vrholder (Autodesk Fusion 360 design; units mm, degrees)
Autodesk Fusion 360 part; units mm, degrees
sketch "Sketch1" plane through (0, 0, 0) normal (1, 0, 0) x (0, 1, 0)
  line L0 (0, 0) -> (0, -40)
  line L1 (0, -40) -> (18.2, -40)
  line L2 (18.2, -40) -> (18.2, 30)
  line L3 (18.2, 30) -> (27.2, 30)
  line L4 (27.2, 30) -> (27.2, 48.65)
  line L5 (33.2, 48.6647) -> (77.2, 48.6647)
  line L6 (77.2, 48.6647) -> (77.2, 68.6647)
  line L7 (27.2, 48.65) -> (7.2, 48.65)
  line L8 (0, 0) -> (-8, 0)
  line L9 (-8, 0) -> (-8, -48)
  line L10 (-8, -48) -> (24.2, -48)
  line L11 (24.2, -48) -> (24.2, 2.6994)
  line L12 (33.2, 22) -> (33.2, 40.6647)
  line L13 (33.2, 40.6647) -> (33.2, 48.6647)
  line L14 (7.2, 48.65) -> (7.2, 54.65)
  line L15 (7.2, 54.65) -> (71.2, 54.65)
  line L16 (71.2, 54.65) -> (71.2, 68.6647)
  line L17 (71.2, 68.6647) -> (77.2, 68.6647)
  line L18 (33.2, 22) -> (24.2, 2.6994)
  line L19 (77.2, 48.6647) -> (24.2, -48)
  line L20 (70.3573, 48.6647) -> (24.2, -35.5199)
  line L21 (33.2, 40.6647) -> (39.2, 48.6647)
  dimension "d1" = 40
  dimension "d2" = 18.2
  dimension "d3" = 70
  dimension "d4" = 9
  dimension "d5" = 18.65
  dimension "d6" = 50
  dimension "d7" = 20
  dimension "d8" = 20
  dimension "d9" = 8
  dimension "d10" = 8
  dimension "d11" = 6
  dimension "d13" = 6
  dimension "d14" = 25
  dimension "d15" = 8
  dimension "d16" = 6
  dimension "d17" = 6
  dimension "d18" = 44
  dimension "d21" = 6
  dimension "d22" = 6
  dimension "d23" = 8
  constraint coincident L0.start L8.start
  constraint vertical L0
  constraint perpendicular L0 L1
  constraint perpendicular L1 L2
  constraint perpendicular L2 L3
  constraint perpendicular L3 L4
  constraint perpendicular L4 L5
  constraint perpendicular L5 L6
  constraint perpendicular L4 L7
  constraint perpendicular L0 L8
  constraint perpendicular L8 L9
  constraint perpendicular L0 L10
  constraint perpendicular L10 L11
  constraint perpendicular L5 L13
  constraint perpendicular L7 L14
  constraint perpendicular L14 L15
  constraint perpendicular L15 L16
  constraint parallel L5 L17
  constraint coincident L5 L20.start
  constraint coincident L11 L20.end
  constraint parallel L19 L20
  constraint coincident L5 L21.end
  measures "d1" distance of L0.start L0.end
  measures "d2" distance of L0.end L1.end
  measures "d3" distance of L1.end L2.end
  measures "d4" distance of L2.end L3.end
  measures "d5" distance of L3.end L4.end
  measures "d6" distance of L4.end L5.end
  measures "d7" distance of L5.end L6.end
  measures "d8" distance of L4.end L7.end
  measures "d9" distance of L0.start L8.end
  measures "d10" distance of L1 L10
  measures "d11" distance of L2 L11
  measures "d13" distance of L4 L12
  measures "d14" angle of L11 L18
  measures "d15" distance of L3 L12.start
  measures "d16" distance of L7.end L14.end
  measures "d17" distance of L6.end L16.end
  measures "d18" distance of L5.end L5.start
  measures "d21" distance of L19 L20
  measures "d22" distance of L5.start L21.end
  measures "d23" distance of L12.end L5.start
extrude "Extrude1" add sketch "Sketch1" along normal blind 22 contours L0 L1 L2 L3 L4 L5 L6 L7 L8 L9 L10 L11 L12 L13 L14 L15 L16 L17 L18 | L5 L11 L19 L20 | L5 L13 L21
